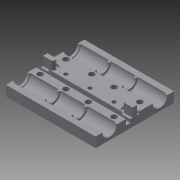
# Autodesk Inventor part: bart xl dual extruder x carriage v6 front
Saved by Autodesk Inventor 2014 SP1 (Build 180222100, 222)
## iProperties
Created: 2015-07-20
Part Number: bart xl dual extruder x carriage v6 front
Material: Generic
Document SubType Name: Modeling
Designer: Mon
Density: 1 g/cm^3
Appearance: Default
Author: Mon
Autodesk Inventor part; units mm, degrees
ref_plane "YZ Plane" through (0, 0, 0) normal (1, 0, 0) x (0, 1, 0)
sketch "Sketch1" plane through (0, 0, 0) normal (0, 0, 1) x (1, 0, 0)
  line L0 (0, 0) -> (80, 0)
  line L1 (80, 0) -> (80, 70)
  line L2 (80, 70) -> (0, 70)
  line L3 (0, 70) -> (0, 0)
  line L4 (-55.3096, 35) -> (212.1853, 35)
  line L5 (-55.3096, 35) -> (-55.3096, 56) construction
  line L6 (-55.3096, 56) -> (228.4464, 56)
  line L7 (-55.3096, 35) -> (-55.3096, 14) construction
  line L8 (-55.3096, 14) -> (197.431, 14)
  line L9 (40, 94.4417) -> (40, -29.193)
  line L10 (40, 35) -> (45, 35) construction
  line L11 (40, 50.2474) -> (50, 50.2474) construction
  line L12 (50, 50.2474) -> (50, -10.3935) construction
  line L13 (40, 50.2474) -> (30, 50.2474) construction
  line L14 (30, 50.2474) -> (30, 3.7445) construction
  line L15 (50, 35) -> (73, 35) construction
  line L16 (73, 35) -> (73, 23.5) construction
  line L17 (73, 23.5) -> (7, 23.5) construction
  line L18 (7, 23.5) -> (7, 46.5) construction
  line L19 (7, 46.5) -> (73, 46.5) construction
  line L20 (73, 46.5) -> (73, 35) construction
  circle A0 centre (7, 23.5) radius 2.5
  circle A1 centre (7, 46.5) radius 2.5
  circle A2 centre (73, 46.5) radius 2.5
  circle A3 centre (73, 23.5) radius 2.5
  circle A4 centre (50, 23.5) radius 2.5
  circle A5 centre (50, 46.5) radius 2.5
  circle A6 centre (30, 46.5) radius 2.5
  circle A7 centre (30, 23.5) radius 2.5
  dimension "d0" = 80
  dimension "d1" = 70
  dimension "d2" = 21
  dimension "d3" = 21
  dimension "d39" = 10
  dimension "d40" = 10
  dimension "d41" = 23
  dimension "d42" = 11.5
  dimension "d43" = 66
  dimension "d44" = 23
  dimension "d45" = 66
  dimension "d46" = 11.5
  dimension "d47" = 5
  dimension "d48" = 5
  dimension "d49" = 5
  dimension "d50" = 5
  dimension "d51" = 5
  dimension "d52" = 5
  dimension "d53" = 5
  dimension "d54" = 5
  constraints: 42 end point, 15 point on line, 12 perpendicular, 8 centre point, 4 coincident, 4 parallel, 1 horizontal
  measures "d0" distance of L2.end L1.end
  measures "d1" distance of L1.end L0.end
  measures "d2" distance of L4.start L5.end
  measures "d3" distance of L4.start L7.end
  measures "d39" distance of L11.start L11.end
  measures "d40" distance of L11.start L13.end
  measures "d41" distance of L15.start L15.end
  measures "d42" distance of L15.end L16.end
  measures "d43" distance of L16.end L17.end
  measures "d44" distance of L17.end L18.end
  measures "d45" distance of L18.end L19.end
  measures "d46" distance of L19.end L15.end
  measures "d47" diameter of A0
  measures "d48" diameter of A1
  measures "d49" diameter of A2
  measures "d50" diameter of A3
  measures "d51" diameter of A4
  measures "d52" diameter of A5
  measures "d53" diameter of A6
  measures "d54" diameter of A7
extrude "Extrusion4" add sketch "Sketch1" against normal blind 14
sketch "Sketch4" plane through (80, 0, 0) normal (1, 0, 0) x (0, 0, -1)
  line L0 (0, 0) -> (0, 70) projected
  line L1 (0, 70) -> (14, 70) projected
  line L2 (-9.1612, 35) -> (23.3912, 35) construction
  line L3 (7.115, 74.6265) -> (7.115, -4.7415) construction
  line L4 (-9.1612, 35) -> (-9.1612, 57.5) construction
  line L5 (-9.1612, 57.5) -> (25.0016, 57.5) construction
  line L6 (25.0016, 57.5) -> (25.0016, 12.5) construction
  line L7 (25.0016, 12.5) -> (-9.8513, 12.5) construction
  circle A0 centre (0, 57.5) radius 7.5
  dimension "d57" = 22.5
  dimension "d58" = 45
  dimension "d59" = 15
  constraints: 12 end point, 4 parallel, 2 perpendicular, 2 point on line, 1 centre point
  measures "d57" distance of L2.start L4.end
  measures "d58" distance of L5.end L6.end
  measures "d59" diameter of A0
extrude "Extrusion5" cut sketch "Sketch4" against normal through all
sketch "Sketch5" plane through (80, 0, -14) normal (1, 0, 0) x (0, 0, -1)
  line L0 (-14, 0) -> (-14, 50) projected
  circle A0 centre (-14, 12.5124) radius 7.5
  dimension "d62" = 15
  constraints: 1 centre point, 1 point on line
  measures "d62" diameter of A0
extrude "Extrusion6" cut sketch "Sketch5" against normal through all
sketch "Sketch7" plane through (80, 0, -14) normal (1, 0, 0) x (0, 0, -1)
  arc A0 (-14, 50) -> (-14, 65) centre (-14, 57.5) ccw projected
  line L0 (-14, 20.0124) -> (-14, 50) projected
  arc A1 (-14, 51) -> (-14, 64) centre (-14, 57.5) ccw
  line L1 (-14, 65) -> (-14, 64)
  line L2 (-14, 51) -> (-14, 50)
  constraints: 4 end point, 3 point on circle, 2 collinear, 1 centre point, 1 coincident
extrude "Extrusion7" add sketch "Sketch7" against normal blind 2
sketch "Sketch8" plane through (80, 0, -14) normal (1, 0, 0) x (0, 0, -1)
  arc A0 (-14, 5.0124) -> (-14, 20.0124) centre (-14, 12.5124) ccw projected
  line L0 (-14, 51) -> (-14, 20.0124) projected
  arc A1 (-14, 6.0124) -> (-14, 19.0124) centre (-14, 12.5124) ccw
  line L1 (-14, 20.0124) -> (-14, 19.0124)
  line L2 (-14, 6.0124) -> (-14, 5.0124)
  dimension "d74" = 13
  constraints: 4 end point, 2 collinear, 2 point on circle, 1 centre point, 1 coincident
  measures "d74" diameter of A1
extrude "Extrusion8" add sketch "Sketch8" against normal blind 2
sketch "Sketch9" plane through (0, 0, -14) normal (-1, 0, 0) x (0, 0, 1)
  arc A0 (14, 65) -> (14, 50) centre (14, 57.5) ccw projected
  line L0 (14, 5.0124) -> (14, 0) projected
  arc A1 (14, 64) -> (14, 51) centre (14, 57.5) ccw
  line L1 (14, 65) -> (14, 64)
  line L2 (14, 51) -> (14, 50)
  dimension "d77" = 13
  constraints: 4 end point, 2 collinear, 2 point on circle, 1 centre point, 1 coincident
  measures "d77" diameter of A1
extrude "Extrusion9" add sketch "Sketch9" against normal blind 2
sketch "Sketch10" plane through (0, 0, -14) normal (-1, 0, 0) x (0, 0, 1)
  arc A0 (14, 20.0124) -> (14, 5.0124) centre (14, 12.5124) ccw projected
  line L0 (14, 5.0124) -> (14, 0) projected
  arc A1 (14, 19.0124) -> (14, 6.0124) centre (14, 12.5124) ccw
  line L1 (14, 20.0124) -> (14, 19.0124)
  line L2 (14, 6.0124) -> (14, 5.0124)
  dimension "d80" = 13
  constraints: 4 end point, 2 collinear, 2 point on circle, 1 centre point, 1 coincident
  measures "d80" diameter of A1
extrude "Extrusion10" add sketch "Sketch10" against normal blind 2
ref_plane "Work Plane1" through (51, 0, -14) normal (1, 0, 0) x (0, 0, -1)
sketch "Sketch11" plane through (51, 0, -14) normal (1, 0, 0) x (0, 0, -1)
  arc A0 (-13.9261, 7.0005) -> (-13.998, 18) centre (-14, 12.5) ccw
  line L0 (-13.998, 19.9561) -> (-13.998, 18)
  line L1 (-13.9261, 7.0005) -> (-13.9261, 4.9561)
  point P0 (-14, 0)
  dimension "d84" = 11
  constraints: 4 end point, 2 point on circle, 1 centre point, 1 parallel
  measures "d84" diameter of A0
extrude "Extrusion11" add sketch "Sketch11" along normal blind 2 fills toward (-13.8761, 5.9783) open curves L1 A0 L0
ref_plane "Work Plane4" through (27, 0, -14) normal (-1, 0, 0) x (0, 0, 1)
sketch "Sketch14" plane through (51, 0, -14) normal (1, 0, 0) x (0, 0, -1)
  line L0 (-14, 50) -> (-14, 52)
  arc A0 (-14, 52) -> (-14, 63) centre (-14, 57.5) ccw
  line L1 (-14, 63) -> (-14, 65)
  arc A1 (-14, 50.067) -> (-14, 64.933) centre (-14, 57.5) ccw
  point P0 (-14, 0)
  constraints: 4 end point, 4 point on circle, 2 centre point, 2 point on line, 1 coincident
extrude "Extrusion13" add sketch "Sketch14" along normal blind 2
sketch "Sketch15" plane through (27, 0, -14) normal (-1, 0, 0) x (0, 0, 1)
  line L0 (14, 20) -> (14, 18)
  arc A0 (14, 18) -> (14, 7) centre (14, 12.5) ccw
  arc A1 (14, 20) -> (14, 5) centre (14, 12.5) ccw
  line L1 (14, 7) -> (14, 5)
  point P0 (14, 0)
  dimension "d99" = 11
  dimension "d100" = 15
  constraints: 4 end point, 4 point on circle, 2 centre point, 1 coincident
  measures "d99" diameter of A0
  measures "d100" diameter of A1
extrude "Extrusion14" add sketch "Sketch15" against normal blind 2
sketch "Sketch16" plane through (27, 0, -14) normal (-1, 0, 0) x (0, 0, 1)
  line L0 (14, 65) -> (14, 63)
  arc A0 (14, 63) -> (14, 52) centre (14, 57.5) ccw
  arc A1 (14, 65) -> (14, 50) centre (14, 57.5) ccw
  line L1 (14, 52) -> (14, 50)
  point P0 (14, 0)
  dimension "d103" = 11
  dimension "d104" = 15
  constraints: 4 end point, 4 point on circle, 2 centre point, 1 coincident
  measures "d103" diameter of A0
  measures "d104" diameter of A1
extrude "Extrusion15" add sketch "Sketch16" against normal blind 2
sketch "Sketch17" plane through (80, 0, -14) normal (1, 0, 0) x (0, 0, -1)
  line L0 (-14, 0) -> (0, 0) projected
  line L1 (0, 70) -> (-5, 70)
  line L2 (-5, 70) -> (-5, 0)
  line L3 (-5, 0) -> (0, 0)
  line L4 (0, 0) -> (0, 70)
  constraints: 8 end point, 2 parallel, 1 horizontal, 1 perpendicular, 1 point on line
extrude "Extrusion16" cut sketch "Sketch17" against normal through all
sketch "Sketch18" plane through (80, 0, -9) normal (0, 0, -1) x (-1, 0, 0)
  line L0 (80, 0) -> (0, 0) projected
  circle A0 centre (73, 23.5) radius 2.5 projected
  circle A1 centre (73, 46.5) radius 2.5 projected
  circle A2 centre (7, 46.5) radius 2.5 projected
  circle A3 centre (7, 23.5) radius 2.5 projected
  circle A4 centre (50, 46.5) radius 2.5 projected
  circle A5 centre (50, 23.5) radius 2.5 projected
  circle A6 centre (30, 23.5) radius 2.5 projected
  circle A7 centre (30, 46.5) radius 2.5 projected
  line L1 (7, 46.5) -> (30, 23.5) construction
  line L2 (30, 23.5) -> (50, 46.5) construction
  line L3 (50, 46.5) -> (73, 23.5) construction
  line L4 (73, 23.5) -> (73, 46.5) construction
  line L5 (73, 46.5) -> (50, 23.5) construction
  line L6 (50, 23.5) -> (30, 46.5) construction
  line L7 (30, 46.5) -> (7, 23.5) construction
  point P0 (18.5, 35)
  point P1 (40, 35)
  point P2 (61.5, 35)
  constraints: 14 end point, 3 midpoint, 2 parallel, 2 perpendicular
hole "Hole2" at (61.5, 35, -9) at (40, 35, -9) at (18.5, 35, -9) direction (0, 0, 1) diameter 3.5 end through all counterbore diameter 6 counterbore depth 4
sketch "Sketch25" plane through (0, 0, 0) normal (0, 0, 1) x (1, 0, 0)
  circle A0 centre (61.5, 35) radius 1.75 projected
  line L0 (80, 51) -> (80, 19.0124) projected
  line L1 (78, 50) -> (29, 50) projected
  line L2 (2, 20.0124) -> (2, 19.0124) projected
  line L3 (73, 50) -> (73, 18) construction
  line L4 (61.5, 35) -> (92.4845, 35) construction
  arc A1 (73, 39) -> (73, 31) centre (73, 35) ccw
  arc A2 (73, 37) -> (73, 33) centre (73, 35) ccw
  line L5 (73, 39) -> (80, 39)
  line L6 (80, 37) -> (73, 37)
  line L7 (73, 33) -> (80, 33)
  line L8 (80, 31) -> (73, 31)
  point P0 (0, 0)
  constraints: 12 end point, 11 point on line, 4 point on circle, 4 tangent, 3 parallel, 3 perpendicular, 2 centre point, 1 coincident
extrude "Extrusion23" cut sketch "Sketch25" against normal blind 2 contours L0 L6 A2 L7 L8 A1 L5
sketch "Sketch26" plane through (0, 0, 0) normal (0, 0, 1) x (1, 0, 0)
  line L0 (0, 19.0124) -> (0, 51) projected
  circle A0 centre (7, 23.5) radius 2.5 projected
  circle A1 centre (7, 46.5) radius 2.5 projected
  circle A2 centre (18.5, 35) radius 1.75 projected
  line L1 (18.5, 35) -> (-4, 35) construction
  line L2 (7, 46.5) -> (7, 23.5) construction
  arc A3 (7, 33) -> (7, 37) centre (7, 35) ccw
  arc A4 (7, 31) -> (7, 39) centre (7, 35) ccw
  line L3 (7, 39) -> (0, 39)
  line L4 (0, 37) -> (7, 37)
  line L5 (7, 33) -> (0, 33)
  line L6 (0, 31) -> (7, 31)
  point P0 (0, 0)
  constraints: 12 end point, 8 point on line, 5 point on circle, 3 perpendicular, 3 tangent, 2 centre point, 2 parallel, 1 coincident, 1 midpoint
extrude "Extrusion24" cut sketch "Sketch26" against normal blind 2 contours L0 L5 A3 L4 L3 A4 L6
sketch "Sketch27" plane through (0, 0, 0) normal (0, 0, 1) x (1, 0, 0)
  line L0 (73, 33) -> (80, 33) projected
  arc A0 (73, 37) -> (73, 33) centre (73, 35) ccw projected
  arc A1 (73, 37) -> (73, 33) centre (73, 35) ccw
  line L1 (80, 37) -> (73, 37)
  line L2 (73, 33) -> (80, 33)
  line L3 (80, 33) -> (80, 37)
  point P0 (0, 0)
  constraints: 6 end point, 2 point on circle, 1 centre point, 1 coincident, 1 horizontal, 1 parallel, 1 point on line
extrude "Extrusion25" add sketch "Sketch27" along normal blind 6
sketch "Sketch28" plane through (0, 0, 0) normal (0, 0, 1) x (1, 0, 0)
  arc A0 (7, 33) -> (7, 37) centre (7, 35) ccw projected
  arc A1 (7, 33) -> (7, 37) centre (7, 35) ccw
  line L0 (0, 37) -> (7, 37)
  line L1 (7, 33) -> (0, 33)
  line L2 (0, 33) -> (0, 37)
  point P0 (0, 0)
  constraints: 6 end point, 2 point on circle, 1 centre point, 1 coincident, 1 concentric, 1 horizontal, 1 parallel
extrude "Extrusion26" add sketch "Sketch28" along normal blind 6
sketch "Sketch29" plane through (0, 0, 0) normal (0, 0, 1) x (1, 0, 0)
  line L0 (80, 31) -> (80, 19.0124) projected
  line L1 (0, 31) -> (80, 31)
  line L2 (80, 31) -> (80, 27)
  line L3 (80, 27) -> (0, 27)
  line L4 (0, 27) -> (0, 31)
  point P0 (0, 0)
  constraints: 8 end point, 2 parallel, 1 horizontal, 1 perpendicular, 1 point on line
extrude "Extrusion27" cut sketch "Sketch29" against normal blind 5
body "Solid2"
